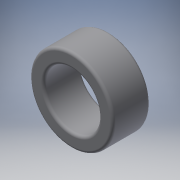
# Autodesk Inventor part: guma
Saved by Autodesk Inventor 2016 (Build 200138000, 138)
## iProperties
Created: 2016-11-29
Part Number: guma
Material: Generic
Document SubType Name: Modeling
Designer: Juraj
Density: 1 g/cm^3
Appearance: Default
Author: Juraj
Autodesk Inventor part; units mm, degrees
ref_plane "YZ Plane" through (0, 0, 0) normal (1, 0, 0) x (0, 1, 0)
ref_plane "XZ Plane" through (0, 0, 0) normal (0, 1, 0) x (-1, 0, 0)
ref_plane "XY Plane" through (0, 0, 0) normal (0, 0, 1) x (1, 0, 0)
sketch "Sketch1" plane through (0, 0, 0) normal (0, 1, 0) x (-1, 0, 0)
  circle A0 centre (0, 0) radius 29.25
  circle A1 centre (0, 0) radius 44.25
  dimension "d0" = 58.5
  dimension "d1" = 15
  constraints: 2 centre point, 2 coincident
  measures "d0" diameter of A0
  measures "d1" radial gap between concentric circles of A1 A0
extrude "Extrusion1" add sketch "Sketch1" along normal blind 40
fillet "Fillet1" radius 3 2 edges at (44.25, 40, 0) (44.25, 0, 0)
fillet "Fillet2" radius 3 2 edges at (29.25, 40, 0) (29.25, 0, 0)
body "Solid1"
